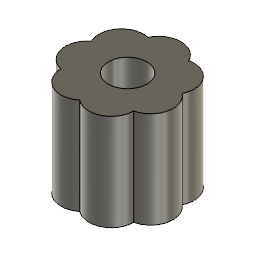
knob (Autodesk Fusion 360 design; units mm, degrees)
Autodesk Fusion 360 part; units mm, degrees
sketch "Sketch2" plane through (0, 0, 0) normal (0, 0, 1) x (1, 0, 0)
  circle A0 centre (0, 0) radius 8.5
  circle A1 centre (0, 0) radius 3
  circle A2 centre (0, 5) radius 3.5
  circle A3 centre (-3.9092, 3.1174) radius 3.5
  circle A4 centre (-4.8746, -1.1126) radius 3.5
  circle A5 centre (-2.1694, -4.5048) radius 3.5
  circle A6 centre (2.1694, -4.5048) radius 3.5
  circle A7 centre (4.8746, -1.1126) radius 3.5
  circle A8 centre (3.9092, 3.1174) radius 3.5
  dimension "d3" = 17
  dimension "d5" = 6
  dimension "d6" = 7
  dimension "d8" = 360
  constraint coincident A0.centre A1.centre
  constraint concentric A0 A1
  measures "d3" diameter of A0
  measures "d5" diameter of A1
  measures "d6" diameter of A2
extrude "Extrude1" add sketch "Sketch2" along normal blind 9 contours A1 A2 A7 A8 | A1 A2 A3 A8 | A1 A2 A8 | A1 A2 A3 A4 | A1 A2 A3 | A1 A7 A8 | A1 A6 A7 A8 | A1 A2 A3 A8 | A1 A2 A8 | A1 A3 A4 A5 | A1 A3 A4 | A1 A2 A3 A4 | A1 A2 A3 | A1 A2 A7 A8 | A1 A7 A8 | A1 A6 A7 A8 | A2 A3 A4 A5 A6 A7 A8 | A1 A4 A5 A6 | A1 A4 A5 | A1 A3 A4 A5 | A1 A3 A4 | A1 A6 A7 | A1 A6 A7 | A1 A5 A6 A7 | A1 A5 A6 | A1 A4 A5 A6 | A1 A4 A5 | A1 A5 A6 A7 | A1 A5 A6
extrude "Extrude2" add 1 faces at (1.3078, 0.2985, 9) along direction (0, 0, 1) blind 6
hole "Hole1" at (0.0633, 0.1229, 15) direction (0, 0, -1) diameter 6 depth 11 tip angle 180
